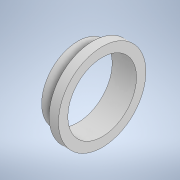
# Autodesk Inventor part: 轴套3
Saved by Autodesk Inventor 2020 (Build 240168000, 168)
## iProperties
Created: 2021-06-17
Part Number: 轴套3
Material: 常规
Document SubType Name: Modeling
Designer: dell
Density: 1 g/cm^3
Appearance: 默认
Author: dell
Autodesk Inventor part; units mm, degrees
ref_plane "YZ Plane" through (0, 0, 0) normal (1, 0, 0) x (0, 1, 0)
ref_plane "XZ Plane" through (0, 0, 0) normal (0, 1, 0) x (-1, 0, 0)
ref_plane "XY Plane" through (0, 0, 0) normal (0, 0, 1) x (1, 0, 0)
sketch "草图1" plane through (0, 0, 0) normal (0, 0, 1) x (1, 0, 0)
  line L0 (0, -98) -> (0, 98) construction
  line L1 (-46.8, 0) -> (7.8, 0) construction
  line L2 (-39, 58) -> (-15, 58)
  line L3 (-15, -58) -> (-39, -58)
  line L4 (-39, -58) -> (-39, 58)
  line L5 (-39, 55) -> (-39, 55)
  line L6 (-39, -55) -> (-39, -55)
  line L7 (-39, -55) -> (-39, 55)
  line L8 (-15, 70) -> (0, 70)
  line L9 (0, 70) -> (0, -70)
  line L10 (0, -70) -> (-15, -70)
  line L11 (-15, -70) -> (-15, -58)
  line L12 (-15, 58) -> (-15, 70)
  line L13 (-39, 55) -> (0, 55)
  line L14 (-39, -55) -> (0, -55)
  point P0 (0, 0)
  dimension "d0" = 140
  dimension "d1" = 110
  dimension "d2" = 39
  dimension "d3" = 15
  dimension "d4" = 116
  constraints: 26 end point, 5 parallel, 5 point on line, 4 horizontal, 2 perpendicular, 1 collinear, 1 midpoint, 2 other
  measures "d0" distance between parallel lines of L10 L8
  measures "d1" distance between parallel lines of L14 L13
  measures "d2" distance between parallel lines of L9 L4
  measures "d3" distance between parallel lines of L9 L12
  measures "d4" distance between parallel lines of L3 L2
revolve "旋转1" add sketch "草图1" angle 360 about axis through (-10, 0, 0) along (1, 0, 0) contours L2 L12 L8 L9 L13 L4
